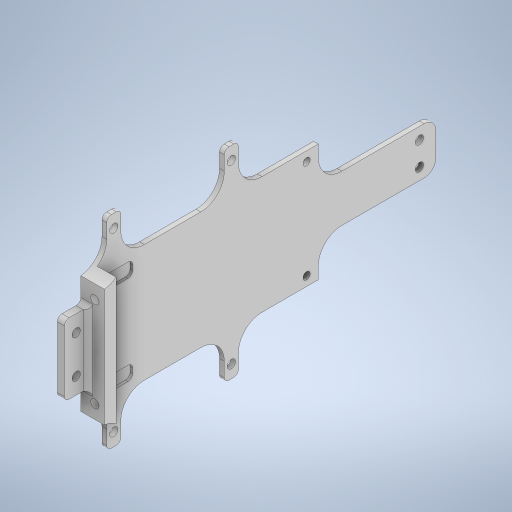
# Autodesk Inventor part: POUPLY_P3_batterie_support_V2
Saved by Autodesk Inventor 2024 (Build 280153000, 153)
## iProperties
Created: 2024-04-03
Part Number: POUPLY_P3_batterie_support_V2
Material: Generic
Document SubType Name: Modeling
Designer: luc4s
Density: 1 g/cm^3
Appearance: Default
Author: luc4s
## iProperties of the stored document POUPLY_P3_batterie_support_V2_3DPrint.ipt
Created: 2024-04-05
Part Number: POUPLY_P3_batterie_support_V2_3DPrint
Material: Generic
Document SubType Name: Modeling
Designer: luc4s
Density: 1 g/cm^3
Appearance: Default
Author: luc4s
Autodesk Inventor part; units mm, degrees
ref_plane "YZ Plane" through (0, 0, 0) normal (1, 0, 0) x (0, 1, 0)
ref_plane "XZ Plane" through (0, 0, 0) normal (0, 1, 0) x (-1, 0, 0)
ref_plane "XY Plane" through (0, 0, 0) normal (0, 0, 1) x (1, 0, 0)
sketch "Sketch1" plane through (0, 0, 0) normal (1, 0, 0) x (0, 1, 0)
  line L0 (25, 49.5) -> (-25, 49.5)
  line L1 (-25, 49.5) -> (-25, -49.5)
  line L2 (-25, -49.5) -> (25, -49.5)
  line L3 (25, -49.5) -> (25, 49.5)
  line L4 (0, 49.5) -> (0, -49.5) construction
  line L5 (25, 0) -> (-25, 0) construction
  point P0 (0, 0)
  dimension "d0" = 99
  dimension "d1" = 50
  constraints: 12 end point, 6 midpoint, 2 parallel, 1 horizontal, 1 perpendicular
  measures "d0" distance of L2.end L0.start
  measures "d1" distance of L0.start L0.end
extrude "Extrusion1" add sketch "Sketch1" along normal blind 2
sketch "Sketch6" plane through (2, 0, 0) normal (1, 0, 0) x (0, 0, -1)
  circle A0 centre (44.5, 21) radius 1.5
  line L0 (49.5, -25) -> (49.5, 25) projected
  line L1 (49.5, 25) -> (-49.5, 25) projected
  point P0 (0, 0)
  dimension "d21" = 3
  dimension "d22" = 5
  dimension "d23" = 4
  constraints: 1 centre point
  measures "d21" diameter of A0
  measures "d22" distance from line of L0 A0.centre
  measures "d23" distance from line of L1 A0.centre
sketch "Sketch7" plane through (2, 0, 0) normal (1, 0, 0) x (0, 0, -1)
  line L0 (49.5, 25) -> (-49.5, 25) projected
  line L1 (-49.5, -25) -> (49.5, -25) projected
  line L2 (-49.5, 25) -> (-44.5, 25)
  line L3 (-44.5, 25) -> (-44.5, -25)
  line L4 (-44.5, -25) -> (-49.5, -25)
  line L5 (-49.5, -25) -> (-49.5, 25)
  point P0 (0, 0)
  dimension "d26" = 5
  constraints: 8 end point, 2 parallel, 1 horizontal, 1 perpendicular, 1 point on line
  measures "d26" distance between parallel lines of L3 L5
extrude "Extrusion6" add sketch "Sketch7" along normal blind 8
sketch "Sketch9" plane through (2, 0, 0) normal (1, 0, 0) x (0, 0, -1)
  line L0 (-44.5, -25) -> (-44.5, 25) projected
  line L1 (-44.5, -22) -> (-29.5, -22)
  line L2 (-29.5, -22) -> (-29.5, -16)
  line L3 (-29.5, -16) -> (-44.5, -16)
  line L4 (-44.5, -16) -> (-44.5, -22)
  line L5 (-44.5, -25) -> (49.5, -25) projected
  point P0 (0, 0)
  point P1 (-37, -22)
  dimension "d34" = 6
  dimension "d35" = 3
  dimension "d36" = 15
  constraints: 8 end point, 2 parallel, 1 horizontal, 1 midpoint, 1 perpendicular, 1 point on line
  measures "d34" distance of L1.end L2.end
  measures "d35" distance from line of L5 point (-37, -22)
  measures "d36" distance of L2.end L3.end
extrude "Extrusion8" cut sketch "Sketch9" against normal blind 1
fillet "Fillet1" radius 2 2 edges at (1.5, -22, 29.5) (1.5, -16, 29.5)
mirror "Mirror3" about plane through (0, 0, 0) normal (0, 1, 0) of "Extrusion8", "Fillet1"
extrude "Extrusion9" cut sketch "Sketch6" against normal blind 10
mirror "Mirror4" about plane through (0, 0, 0) normal (0, 1, 0) of "Extrusion9"
sketch "Sketch11" plane through (0, 0, 0) normal (-1, 0, 0) x (0, 0, 1)
  line L0 (40.5, -25) -> (34.5, -25)
  line L1 (34.5, -25) -> (34.5, -43)
  line L2 (34.5, -43) -> (40.5, -43)
  line L3 (40.5, -43) -> (40.5, -25)
  line L4 (49.5, -25) -> (-49.5, -25) projected
  line L5 (49.5, 25) -> (49.5, -25) projected
  point P0 (0, 0)
  dimension "d45" = 18
  dimension "d46" = 6
  dimension "d47" = 15
  constraints: 8 end point, 2 parallel, 1 horizontal, 1 perpendicular, 1 point on line
  measures "d45" distance of L0.end L1.end
  measures "d46" distance of L1.end L2.end
  measures "d47" distance from line of L5 L0.end
extrude "Extrusion10" add sketch "Sketch11" against normal blind 2
mirror "Mirror5" about plane through (0, 0, 0) normal (0, 1, 0) of "Extrusion10"
sketch "Sketch12" plane through (0, 0, 0) normal (-1, 0, 0) x (0, 0, 1)
  circle A0 centre (37.5, -37.5) radius 1.75
  line L0 (34.5, -25) -> (-49.5, -25) projected
  line L1 (40.5, -43) -> (40.5, -25) projected
  point P0 (0, 0)
  dimension "d50" = 12.5
  dimension "d51" = 3
  dimension "d52" = 3.5
  constraints: 1 centre point
  measures "d50" distance from line of L0 A0.centre
  measures "d51" distance from line of L1 A0.centre
  measures "d52" diameter of A0
extrude "Extrusion11" cut sketch "Sketch12" against normal blind 2
mirror "Mirror6" about plane through (0, 0, 0) normal (0, 1, 0) of "Extrusion11"
sketch "Sketch13" plane through (0, -25, 49.5) normal (0, 0, 1) x (1, 0, 0)
  point P0 (0, 25)
sketch "Sketch14" plane through (0, 0, 0) normal (-1, 0, 0) x (0, 0, 1)
  line L0 (49.5, 25) -> (49.5, -25) projected
  line L1 (49.5, 15) -> (59.5, 15)
  line L2 (59.5, 15) -> (59.5, -15)
  line L3 (59.5, -15) -> (49.5, -15)
  line L4 (49.5, -15) -> (49.5, 15)
  point P0 (0, 0)
  dimension "d56" = 30
  dimension "d57" = 10
  dimension "d58" = 10
  constraints: 8 end point, 2 parallel, 1 horizontal, 1 perpendicular, 1 point on line
  measures "d56" distance of L1.end L2.end
  measures "d57" distance from line of L1 L0.start
  measures "d58" distance of L1.start L1.end
extrude "Extrusion12" add sketch "Sketch14" against normal blind 3
chamfer "Chamfer1" distance 2 angle 45 1 edges at (3, 0, 49.5)
fillet "Fillet3" radius 2 6 edges at (1.5, -15, 59.5) (1.5, 15, 59.5) (4, -15, 49.5) (1.5, -15, 49.5) (4, 15, 49.5) (1.5, 15, 49.5)
sketch "Sketch15" plane through (0, 0, 0) normal (-1, 0, 0) x (0, 0, 1)
  circle A0 centre (54.5, -8) radius 1.75
  line L0 (59.5, -13) -> (59.5, 13) projected
  line L1 (51.5, -15) -> (57.5, -15) projected
  point P0 (0, 0)
  dimension "d65" = 3.5
  dimension "d66" = 5
  dimension "d67" = 7
  constraints: 1 centre point
  measures "d65" diameter of A0
  measures "d66" distance from line of L0 A0.centre
  measures "d67" distance from line of L1 A0.centre
extrude "Extrusion13" cut sketch "Sketch15" against normal blind 3
mirror "Mirror7" about plane through (0, 0, 0) normal (0, 1, 0) of "Extrusion13"
pattern_linear "Rectangular Pattern2" count 2 spacing 50 along (0, 0, -1) of "Extrusion10", "Mirror5", "Extrusion11", "Mirror6"
fillet "Fillet4" radius 10 8 edges at (1, -25, -15.5) (1, -25, -9.5) (1, -25, 34.5) (1, -25, 40.5) (1, 25, -15.5) (1, 25, -9.5) (1, 25, 34.5) (1, 25, 40.5)
fillet "Fillet5" radius 2 8 edges at (1, -43, 40.5) (1, -43, 34.5) (1, -43, -9.5) (1, -43, -15.5) (1, 43, 34.5) (1, 43, 40.5) (1, 43, -9.5) (1, 43, -15.5)
sketch "Sketch17" plane through (0, 0, 0) normal (-1, 0, 0) x (0, 0, 1)
  line L0 (-49.5, -25) -> (-49.5, 25) projected
  line L1 (-49.5, -10) -> (-99.5, -10)
  line L2 (-99.5, -10) -> (-99.5, 10)
  line L3 (-99.5, 10) -> (-49.5, 10)
  line L4 (-49.5, 10) -> (-49.5, -10)
  line L5 (-49.5, -25) -> (-49.5, 25) projected
  point P0 (0, 0)
  point P1 (-49.5, 0)
  point P2 (-49.5, 0)
  dimension "d78" = 10
  dimension "d79" = 10
  dimension "d80" = 50
  constraints: 8 end point, 2 midpoint, 2 parallel, 1 horizontal, 1 perpendicular, 1 point on line
  measures "d78" distance from line of point (-49.5, 0) L1
  measures "d79" distance from line of L3 point (-49.5, 0)
  measures "d80" distance of L1.start L1.end
extrude "Extrusion14" add sketch "Sketch17" against normal blind 2
fillet "Fillet6" radius 10 2 edges at (1, 10, -49.5) (1, -10, -49.5)
fillet "Fillet7" radius 5 2 edges at (1, 10, -99.5) (1, -10, -99.5)
sketch "Sketch18" plane through (0, 0, 0) normal (-1, 0, 0) x (0, 0, 1)
  circle A0 centre (-92.5, 5) radius 1.75
  line L0 (-59.5, 10) -> (-94.5, 10) projected
  line L1 (-99.5, 5) -> (-99.5, -5) projected
  point P0 (0, 0)
  dimension "d85" = 3.5
  dimension "d86" = 5
  dimension "d87" = 7
  constraints: 1 centre point
  measures "d85" diameter of A0
  measures "d86" distance from line of L0 A0.centre
  measures "d87" distance from line of L1 A0.centre
extrude "Extrusion15" cut sketch "Sketch18" against normal blind 2
mirror "Mirror8" about plane through (0, 0, 0) normal (0, 1, 0) of "Extrusion15"
sketch "Sketch19" plane through (0, 17, 49.5) normal (0, 0, 1) x (1, 0, 0)
  circle A0 centre (6, 2.15) radius 1.75
  circle A1 centre (6.9195, -35.9182) radius 1.75
  line L0 (10, 8) -> (10, -42) projected
  point P0 (0, -17)
  point P1 (2, 8)
  dimension "d90" = 3.5
  dimension "d91" = 3.5
  dimension "d92" = 4
  dimension "d93" = 5.85
  constraints: 2 centre point
  measures "d90" diameter of A1
  measures "d91" diameter of A0
  measures "d92" distance from line of L0 A0.centre
  measures "d93" vertical distance of point (2, 8) A0.centre
extrude "Extrusion16" cut sketch "Sketch19" against normal blind 10 contours A0
mirror "Mirror9" about plane through (0, 0, 0) normal (0, 1, 0) of "Extrusion16"
body "Solid1"
